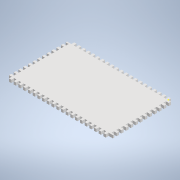
# Autodesk Inventor part: top
Saved by Autodesk Inventor 2022 (Build 260153000, 153)
## iProperties
Created: 2023-05-26
Part Number: top
Material: Типовые
Document SubType Name: Modeling
Designer: korsh624
Density: 1 g/cm^3
Appearance: По умолчанию
Author: korsh624
Autodesk Inventor part; units mm, degrees
ref_plane "YZ Plane" through (0, 0, 0) normal (1, 0, 0) x (0, 1, 0)
ref_plane "XZ Plane" through (0, 0, 0) normal (0, 1, 0) x (-1, 0, 0)
ref_plane "XY Plane" through (0, 0, 0) normal (0, 0, 1) x (1, 0, 0)
sketch "Эскиз1" plane through (0, 0, 0) normal (0, 1, 0) x (-1, 0, 0)
  line L0 (0, 0) -> (208, 0)
  line L1 (208, 0) -> (208, 123)
  line L2 (208, 123) -> (0, 123)
  line L3 (0, 123) -> (0, 0)
  line L4 (208, 125) -> (208, 130)
  line L5 (208, 123) -> (214, 123)
  line L6 (214, 123) -> (214, 118)
  line L7 (214, 118) -> (208, 118)
  line L8 (208, 118) -> (208, 123)
  line L9 (208, 113) -> (214, 113)
  line L10 (214, 113) -> (214, 108)
  line L11 (214, 108) -> (208, 108)
  line L12 (208, 108) -> (208, 113)
  line L13 (208, 103) -> (214, 103)
  line L14 (214, 103) -> (214, 98)
  line L15 (214, 98) -> (208, 98)
  line L16 (208, 98) -> (208, 103)
  line L17 (208, 93) -> (214, 93)
  line L18 (214, 93) -> (214, 88)
  line L19 (214, 88) -> (208, 88)
  line L20 (208, 88) -> (208, 93)
  line L21 (208, 83) -> (214, 83)
  line L22 (214, 83) -> (214, 78)
  line L23 (214, 78) -> (208, 78)
  line L24 (208, 78) -> (208, 83)
  line L25 (208, 73) -> (214, 73)
  line L26 (214, 73) -> (214, 68)
  line L27 (214, 68) -> (208, 68)
  line L28 (208, 68) -> (208, 73)
  line L29 (208, 63) -> (214, 63)
  line L30 (214, 63) -> (214, 58)
  line L31 (214, 58) -> (208, 58)
  line L32 (208, 58) -> (208, 63)
  line L33 (208, 53) -> (214, 53)
  line L34 (214, 53) -> (214, 48)
  line L35 (214, 48) -> (208, 48)
  line L36 (208, 48) -> (208, 53)
  line L37 (208, 43) -> (214, 43)
  line L38 (214, 43) -> (214, 38)
  line L39 (214, 38) -> (208, 38)
  line L40 (208, 38) -> (208, 43)
  line L41 (208, 33) -> (214, 33)
  line L42 (214, 33) -> (214, 28)
  line L43 (214, 28) -> (208, 28)
  line L44 (208, 28) -> (208, 33)
  line L45 (208, 23) -> (214, 23)
  line L46 (214, 23) -> (214, 18)
  line L47 (214, 18) -> (208, 18)
  line L48 (208, 18) -> (208, 23)
  line L49 (208, 13) -> (214, 13)
  line L50 (214, 13) -> (214, 8)
  line L51 (214, 8) -> (208, 8)
  line L52 (208, 8) -> (208, 13)
  line L53 (208, 3) -> (214, 3)
  line L54 (214, 3) -> (214, -2)
  line L55 (214, -2) -> (208, -2)
  line L56 (208, -2) -> (208, 3)
  line L57 (0, 0) -> (-6, 0)
  line L58 (-6, 0) -> (-6, 5)
  line L59 (-6, 5) -> (0, 5)
  line L60 (0, 5) -> (0, 0)
  line L61 (0, 15) -> (0, 10)
  line L62 (0, 10) -> (-6, 10)
  line L63 (-6, 10) -> (-6, 15)
  line L64 (-6, 15) -> (0, 15)
  line L65 (0, 25) -> (0, 20)
  line L66 (0, 20) -> (-6, 20)
  line L67 (-6, 20) -> (-6, 25)
  line L68 (-6, 25) -> (0, 25)
  line L69 (0, 35) -> (0, 30)
  line L70 (0, 30) -> (-6, 30)
  line L71 (-6, 30) -> (-6, 35)
  line L72 (-6, 35) -> (0, 35)
  line L73 (0, 45) -> (0, 40)
  line L74 (0, 40) -> (-6, 40)
  line L75 (-6, 40) -> (-6, 45)
  line L76 (-6, 45) -> (0, 45)
  line L77 (0, 55) -> (0, 50)
  line L78 (0, 50) -> (-6, 50)
  line L79 (-6, 50) -> (-6, 55)
  line L80 (-6, 55) -> (0, 55)
  line L81 (0, 65) -> (0, 60)
  line L82 (0, 60) -> (-6, 60)
  line L83 (-6, 60) -> (-6, 65)
  line L84 (-6, 65) -> (0, 65)
  line L85 (0, 75) -> (0, 70)
  line L86 (0, 70) -> (-6, 70)
  line L87 (-6, 70) -> (-6, 75)
  line L88 (-6, 75) -> (0, 75)
  line L89 (0, 85) -> (0, 80)
  line L90 (0, 80) -> (-6, 80)
  line L91 (-6, 80) -> (-6, 85)
  line L92 (-6, 85) -> (0, 85)
  line L93 (0, 95) -> (0, 90)
  line L94 (0, 90) -> (-6, 90)
  line L95 (-6, 90) -> (-6, 95)
  line L96 (-6, 95) -> (0, 95)
  line L97 (0, 105) -> (0, 100)
  line L98 (0, 100) -> (-6, 100)
  line L99 (-6, 100) -> (-6, 105)
  line L100 (-6, 105) -> (0, 105)
  line L101 (0, 115) -> (0, 110)
  line L102 (0, 110) -> (-6, 110)
  line L103 (-6, 110) -> (-6, 115)
  line L104 (-6, 115) -> (0, 115)
  line L105 (0, 125) -> (0, 120)
  line L106 (0, 120) -> (-6, 120)
  line L107 (-6, 120) -> (-6, 125)
  line L108 (-6, 125) -> (0, 125)
  line L109 (208, 123) -> (203, 123)
  line L110 (203, 123) -> (203, 129)
  line L111 (203, 129) -> (208, 129)
  line L112 (208, 129) -> (208, 123)
  line L113 (198, 125) -> (198, 130)
  line L114 (198, 123) -> (193, 123)
  line L115 (198, 129) -> (198, 123)
  line L116 (193, 129) -> (198, 129)
  line L117 (193, 123) -> (193, 129)
  line L118 (188, 125) -> (188, 130)
  line L119 (188, 123) -> (183, 123)
  line L120 (188, 129) -> (188, 123)
  line L121 (183, 129) -> (188, 129)
  line L122 (183, 123) -> (183, 129)
  line L123 (178, 125) -> (178, 130)
  line L124 (178, 123) -> (173, 123)
  line L125 (178, 129) -> (178, 123)
  line L126 (173, 129) -> (178, 129)
  line L127 (173, 123) -> (173, 129)
  line L128 (168, 125) -> (168, 130)
  line L129 (168, 123) -> (163, 123)
  line L130 (168, 129) -> (168, 123)
  line L131 (163, 129) -> (168, 129)
  line L132 (163, 123) -> (163, 129)
  line L133 (158, 125) -> (158, 130)
  line L134 (158, 123) -> (153, 123)
  line L135 (158, 129) -> (158, 123)
  line L136 (153, 129) -> (158, 129)
  line L137 (153, 123) -> (153, 129)
  line L138 (148, 125) -> (148, 130)
  line L139 (148, 123) -> (143, 123)
  line L140 (148, 129) -> (148, 123)
  line L141 (143, 129) -> (148, 129)
  line L142 (143, 123) -> (143, 129)
  line L143 (138, 125) -> (138, 130)
  line L144 (138, 123) -> (133, 123)
  line L145 (138, 129) -> (138, 123)
  line L146 (133, 129) -> (138, 129)
  line L147 (133, 123) -> (133, 129)
  line L148 (128, 125) -> (128, 130)
  line L149 (128, 123) -> (123, 123)
  line L150 (128, 129) -> (128, 123)
  line L151 (123, 129) -> (128, 129)
  line L152 (123, 123) -> (123, 129)
  line L153 (118, 125) -> (118, 130)
  line L154 (118, 123) -> (113, 123)
  line L155 (118, 129) -> (118, 123)
  line L156 (113, 129) -> (118, 129)
  line L157 (113, 123) -> (113, 129)
  line L158 (108, 125) -> (108, 130)
  line L159 (108, 123) -> (103, 123)
  line L160 (108, 129) -> (108, 123)
  line L161 (103, 129) -> (108, 129)
  line L162 (103, 123) -> (103, 129)
  line L163 (98, 125) -> (98, 130)
  line L164 (98, 123) -> (93, 123)
  line L165 (98, 129) -> (98, 123)
  line L166 (93, 129) -> (98, 129)
  line L167 (93, 123) -> (93, 129)
  line L168 (88, 125) -> (88, 130)
  line L169 (88, 123) -> (83, 123)
  line L170 (88, 129) -> (88, 123)
  line L171 (83, 129) -> (88, 129)
  line L172 (83, 123) -> (83, 129)
  line L173 (78, 125) -> (78, 130)
  line L174 (78, 123) -> (73, 123)
  line L175 (78, 129) -> (78, 123)
  line L176 (73, 129) -> (78, 129)
  line L177 (73, 123) -> (73, 129)
  line L178 (68, 125) -> (68, 130)
  line L179 (68, 123) -> (63, 123)
  line L180 (68, 129) -> (68, 123)
  line L181 (63, 129) -> (68, 129)
  line L182 (63, 123) -> (63, 129)
  line L183 (58, 125) -> (58, 130)
  line L184 (58, 123) -> (53, 123)
  line L185 (58, 129) -> (58, 123)
  line L186 (53, 129) -> (58, 129)
  line L187 (53, 123) -> (53, 129)
  line L188 (48, 125) -> (48, 130)
  line L189 (48, 123) -> (43, 123)
  line L190 (48, 129) -> (48, 123)
  line L191 (43, 129) -> (48, 129)
  line L192 (43, 123) -> (43, 129)
  line L193 (38, 125) -> (38, 130)
  line L194 (38, 123) -> (33, 123)
  line L195 (38, 129) -> (38, 123)
  line L196 (33, 129) -> (38, 129)
  line L197 (33, 123) -> (33, 129)
  line L198 (28, 125) -> (28, 130)
  line L199 (28, 123) -> (23, 123)
  line L200 (28, 129) -> (28, 123)
  line L201 (23, 129) -> (28, 129)
  line L202 (23, 123) -> (23, 129)
  line L203 (18, 125) -> (18, 130)
  line L204 (18, 123) -> (13, 123)
  line L205 (18, 129) -> (18, 123)
  line L206 (13, 129) -> (18, 129)
  line L207 (13, 123) -> (13, 129)
  line L208 (8, 125) -> (8, 130)
  line L209 (8, 123) -> (3, 123)
  line L210 (8, 129) -> (8, 123)
  line L211 (3, 129) -> (8, 129)
  line L212 (3, 123) -> (3, 129)
  line L213 (0, 0) -> (5, 0)
  line L214 (5, 0) -> (5, -6)
  line L215 (5, -6) -> (0, -6)
  line L216 (0, -6) -> (0, 0)
  line L217 (10, 0) -> (15, 0)
  line L218 (10, -6) -> (10, 0)
  line L219 (15, -6) -> (10, -6)
  line L220 (15, 0) -> (15, -6)
  line L221 (20, 0) -> (25, 0)
  line L222 (20, -6) -> (20, 0)
  line L223 (25, -6) -> (20, -6)
  line L224 (25, 0) -> (25, -6)
  line L225 (30, 0) -> (35, 0)
  line L226 (30, -6) -> (30, 0)
  line L227 (35, -6) -> (30, -6)
  line L228 (35, 0) -> (35, -6)
  line L229 (40, 0) -> (45, 0)
  line L230 (40, -6) -> (40, 0)
  line L231 (45, -6) -> (40, -6)
  line L232 (45, 0) -> (45, -6)
  line L233 (50, 0) -> (55, 0)
  line L234 (50, -6) -> (50, 0)
  line L235 (55, -6) -> (50, -6)
  line L236 (55, 0) -> (55, -6)
  line L237 (60, 0) -> (65, 0)
  line L238 (60, -6) -> (60, 0)
  line L239 (65, -6) -> (60, -6)
  line L240 (65, 0) -> (65, -6)
  line L241 (70, 0) -> (75, 0)
  line L242 (70, -6) -> (70, 0)
  line L243 (75, -6) -> (70, -6)
  line L244 (75, 0) -> (75, -6)
  line L245 (80, 0) -> (85, 0)
  line L246 (80, -6) -> (80, 0)
  line L247 (85, -6) -> (80, -6)
  line L248 (85, 0) -> (85, -6)
  line L249 (90, 0) -> (95, 0)
  line L250 (90, -6) -> (90, 0)
  line L251 (95, -6) -> (90, -6)
  line L252 (95, 0) -> (95, -6)
  line L253 (100, 0) -> (105, 0)
  line L254 (100, -6) -> (100, 0)
  line L255 (105, -6) -> (100, -6)
  line L256 (105, 0) -> (105, -6)
  line L257 (110, 0) -> (115, 0)
  line L258 (110, -6) -> (110, 0)
  line L259 (115, -6) -> (110, -6)
  line L260 (115, 0) -> (115, -6)
  line L261 (120, 0) -> (125, 0)
  line L262 (120, -6) -> (120, 0)
  line L263 (125, -6) -> (120, -6)
  line L264 (125, 0) -> (125, -6)
  line L265 (130, 0) -> (135, 0)
  line L266 (130, -6) -> (130, 0)
  line L267 (135, -6) -> (130, -6)
  line L268 (135, 0) -> (135, -6)
  line L269 (140, 0) -> (145, 0)
  line L270 (140, -6) -> (140, 0)
  line L271 (145, -6) -> (140, -6)
  line L272 (145, 0) -> (145, -6)
  line L273 (150, 0) -> (155, 0)
  line L274 (150, -6) -> (150, 0)
  line L275 (155, -6) -> (150, -6)
  line L276 (155, 0) -> (155, -6)
  line L277 (160, 0) -> (165, 0)
  line L278 (160, -6) -> (160, 0)
  line L279 (165, -6) -> (160, -6)
  line L280 (165, 0) -> (165, -6)
  line L281 (170, 0) -> (175, 0)
  line L282 (170, -6) -> (170, 0)
  line L283 (175, -6) -> (170, -6)
  line L284 (175, 0) -> (175, -6)
  line L285 (180, 0) -> (185, 0)
  line L286 (180, -6) -> (180, 0)
  line L287 (185, -6) -> (180, -6)
  line L288 (185, 0) -> (185, -6)
  line L289 (190, 0) -> (195, 0)
  line L290 (190, -6) -> (190, 0)
  line L291 (195, -6) -> (190, -6)
  line L292 (195, 0) -> (195, -6)
  line L293 (200, 0) -> (205, 0)
  line L294 (200, -6) -> (200, 0)
  line L295 (205, -6) -> (200, -6)
  line L296 (205, 0) -> (205, -6)
  point P0 (208, 115)
  point P1 (208, 105)
  point P2 (208, 95)
  point P3 (208, 85)
  point P4 (208, 75)
  point P5 (208, 65)
  point P6 (208, 55)
  point P7 (208, 45)
  point P8 (208, 35)
  point P9 (208, 25)
  point P10 (208, 15)
  point P11 (208, 5)
  point P12 (214, 0)
  point P13 (-6, 123)
  dimension "d9" = 10
  dimension "d15" = 5
  dimension "d18" = 10
  dimension "d27" = 10
  dimension "d36" = 10
  constraints: 586 end point, 200 horizontal alignment, 156 parallel, 128 collinear, 108 vertical alignment, 4 horizontal, 4 perpendicular, 2 point on line, 13 other
  measures "d9" distance of L5.start L9.start
  measures "d15" distance of L57.end L58.end
  measures "d18" distance of L59.end L61.start
  measures "d27" distance of L5.start L114.start
  measures "d36" distance of L213.end L217.end
extrude "Выдавливание1" add sketch "Эскиз1" along normal blind 6 contours L3 L2 L1 L0 | L57 L58 L59 L3 | L0 L214 L215 L216 | L0 L220 L219 L218 | L62 L63 L64 L3 | L66 L67 L68 L3 | L70 L71 L72 L3 | L74 L75 L76 L3 | L78 L79 L80 L3 | L82 L83 L84 L3 | L86 L87 L88 L3 | L90 L91 L92 L3 | L94 L95 L96 L3 | L98 L99 L100 L3 | L102 L103 L104 L3 | L106 L107 L108 L105 L3 | L1 L53 L54 L55 L56 | L1 L49 L50 L51 | L1 L45 L46 L47 | L1 L41 L42 L43 | L1 L37 L38 L39 | L1 L33 L34 L35 | L1 L29 L30 L31 | L1 L25 L26 L27 | L1 L21 L22 L23 | L1 L17 L18 L19 | L1 L13 L14 L15 | L1 L9 L10 L11 | L117 L116 L113 L115 L2 | L1 L5 L6 L7 | L110 L111 L4 L112 L2
sketch "Эскиз2" plane through (0, 6, 0) normal (0, 1, 0) x (1, 0, 0)
  point P0 (0, 0)
